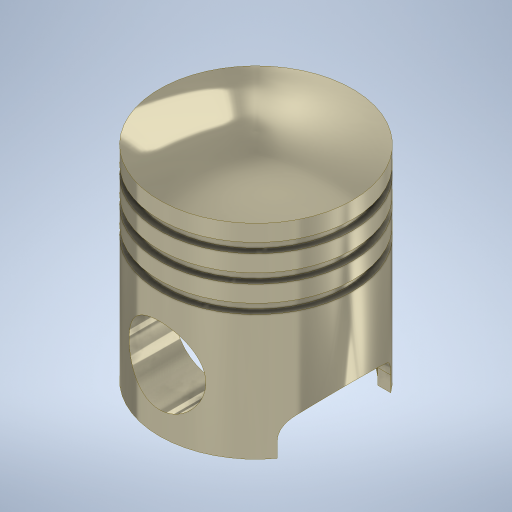
# Autodesk Inventor part: piston
Saved by Autodesk Inventor 2023 (Build 270158000, 158)
## iProperties
Created: 2023-10-20
Part Number: piston
Material: Generic
Document SubType Name: Modeling
Designer: Beatrice
Density: 1 g/cm^3
Appearance: Nickel
Author: Beatrice
Autodesk Inventor part; units mm, degrees
ref_plane "YZ Plane" through (0, 0, 0) normal (1, 0, 0) x (0, 1, 0)
sketch "Sketch1" plane through (0, 0, 0) normal (0, 0, 1) x (1, 0, 0)
  circle A0 centre (0, 0) radius 42.5
  dimension "d0" = 85
  constraints: 1 centre point, 1 coincident
  measures "d0" diameter of A0
extrude "Extrusion1" add sketch "Sketch1" along normal blind 90
ref_plane "Work Plane1" through (0, 0, 82.7) normal (0, 0, 1) x (1, 0, 0)
sketch "Sketch2" plane through (0, 0, 82.7) normal (0, 0, 1) x (1, 0, 0)
  circle A0 centre (0, 0) radius 42.5 projected
  circle A1 centre (0, 0) radius 42.5 projected
  circle A2 centre (0, 0) radius 39.5
  dimension "d4" = 79
  constraints: 3 coincident, 1 centre point
  measures "d4" diameter of A2
extrude "Extrusion2" cut sketch "Sketch2" against normal blind 4.3
pattern_linear "Rectangular Pattern1" count 3 spacing 11.6 along (0, 0, -1) of "Extrusion2"
sketch "Sketch3" plane through (0, 0, 0) normal (0, 0, -1) x (-1, 0, 0)
  circle A0 centre (0, 0) radius 38
  dimension "d10" = 76
  constraints: 1 centre point, 1 coincident
  measures "d10" diameter of A0
hole "Hole1" at (0, 0, 0) direction (0, 0, 1) diameter 76 depth 85
sketch "Sketch4" plane through (0, 0, 0) normal (0, 1, 0) x (-1, 0, 0)
  line L0 (-39.5, 78.4) -> (-39.5, 82.7) construction
  line L1 (-39.5, 82.7) -> (-42.5, 82.7) construction
  line L2 (-42.5, 82.7) -> (-42.5, 90) construction
  line L3 (-42.5, 90) -> (42.5, 90) construction
  line L4 (42.5, 90) -> (42.5, 82.7) construction
  line L5 (42.5, 82.7) -> (39.5, 82.7) construction
  line L6 (39.5, 82.7) -> (39.5, 78.4) construction
  line L7 (39.5, 78.4) -> (42.5, 78.4) construction
  line L8 (42.5, 78.4) -> (42.5, 71.1) construction
  line L9 (42.5, 71.1) -> (39.5, 71.1) construction
  line L10 (39.5, 71.1) -> (39.5, 66.8) construction
  line L11 (39.5, 66.8) -> (42.5, 66.8) construction
  line L12 (42.5, 66.8) -> (42.5, 59.5) construction
  line L13 (42.5, 59.5) -> (39.5, 59.5) construction
  line L14 (39.5, 59.5) -> (39.5, 55.2) construction
  line L15 (39.5, 55.2) -> (42.5, 55.2) construction
  line L16 (42.5, 55.2) -> (42.5, 0) construction
  line L17 (42.5, 0) -> (38, 0) construction
  line L18 (38, 0) -> (38, 85) construction
  line L19 (38, 85) -> (-38, 85) construction
  line L20 (-38, 85) -> (-38, 0) construction
  line L21 (-38, 0) -> (-42.5, 0) construction
  line L22 (-42.5, 0) -> (-42.5, 55.2) construction
  line L23 (-42.5, 55.2) -> (-39.5, 55.2) construction
  line L24 (-39.5, 55.2) -> (-39.5, 59.5) construction
  line L25 (-39.5, 59.5) -> (-42.5, 59.5) construction
  line L26 (-42.5, 59.5) -> (-42.5, 66.8) construction
  line L27 (-42.5, 66.8) -> (-39.5, 66.8) construction
  line L28 (-39.5, 66.8) -> (-39.5, 71.1) construction
  line L29 (-39.5, 71.1) -> (-42.5, 71.1) construction
  line L30 (-42.5, 71.1) -> (-42.5, 78.4) construction
  line L31 (-42.5, 78.4) -> (-39.5, 78.4) construction
  line L32 (0, -18) -> (0, 108) construction
  line L33 (-42.5, 90) -> (0, 90)
  line L34 (0, 90) -> (0, 95)
  line L35 (42.5, 90) -> (-42.5, 90) projected
  arc A0 (0, 95) -> (-42.5, 90) centre (-1.6627, -73.9918) ccw
  line L36 (0, 95) -> (-42.5, 95) construction
  point P0 (0, 0)
  dimension "d18" = 169
  dimension "d19" = 5
  constraints: 6 end point, 2 midpoint, 2 point on circle, 2 point on line, 1 centre point, 1 horizontal, 1 vertical alignment
  measures "d18" radius of A0
  measures "d19" distance of point (0, 90) L34.end
revolve "Revolution1" add sketch "Sketch4" angle 360 about axis through (0, 0, 0) along (0, 0, 1)
sketch "Sketch5" plane through (0, 0, 0) normal (0, 1, 0) x (-1, 0, 0)
  line L0 (-39.5, 78.4) -> (-39.5, 82.7) construction
  line L1 (-39.5, 82.7) -> (-42.5, 82.7) construction
  line L2 (-42.5, 82.7) -> (-42.5, 90) construction
  arc A0 (42.5, 90) -> (0, 95) centre (1.6627, -73.9918) ccw construction
  arc A1 (0, 95) -> (-42.5, 90) centre (-1.6627, -73.9918) ccw construction
  line L3 (42.5, 90) -> (42.5, 82.7) construction
  line L4 (42.5, 82.7) -> (39.5, 82.7) construction
  line L5 (39.5, 82.7) -> (39.5, 78.4) construction
  line L6 (39.5, 78.4) -> (42.5, 78.4) construction
  line L7 (42.5, 78.4) -> (42.5, 71.1) construction
  line L8 (42.5, 71.1) -> (39.5, 71.1) construction
  line L9 (39.5, 71.1) -> (39.5, 66.8) construction
  line L10 (39.5, 66.8) -> (42.5, 66.8) construction
  line L11 (42.5, 66.8) -> (42.5, 59.5) construction
  line L12 (42.5, 59.5) -> (39.5, 59.5) construction
  line L13 (39.5, 59.5) -> (39.5, 55.2) construction
  line L14 (39.5, 55.2) -> (42.5, 55.2) construction
  line L15 (42.5, 55.2) -> (42.5, 0) construction
  line L16 (42.5, 0) -> (38, 0) construction
  line L17 (38, 0) -> (38, 85) construction
  line L18 (38, 85) -> (-38, 85) construction
  line L19 (-38, 85) -> (-38, 0) construction
  line L20 (-38, 0) -> (-42.5, 0) construction
  line L21 (-42.5, 0) -> (-42.5, 55.2) construction
  line L22 (-42.5, 55.2) -> (-39.5, 55.2) construction
  line L23 (-39.5, 55.2) -> (-39.5, 59.5) construction
  line L24 (-39.5, 59.5) -> (-42.5, 59.5) construction
  line L25 (-42.5, 59.5) -> (-42.5, 66.8) construction
  line L26 (-42.5, 66.8) -> (-39.5, 66.8) construction
  line L27 (-39.5, 66.8) -> (-39.5, 71.1) construction
  line L28 (-39.5, 71.1) -> (-42.5, 71.1) construction
  line L29 (-42.5, 71.1) -> (-42.5, 78.4) construction
  line L30 (-42.5, 78.4) -> (-39.5, 78.4) construction
  line L31 (0, -108.0603) -> (0, 130.4191) construction
  circle A2 centre (0, 27) radius 16.9
  point P0 (0, 0)
  dimension "d21" = 33.8
  dimension "d22" = 27
  constraints: 1 centre point, 1 point on line
  measures "d21" diameter of A2
  measures "d22" vertical distance of L16.end A2.centre
extrude "Extrusion3" cut sketch "Sketch5" along normal through all both and the other way through all
sketch "Sketch6" plane through (0, 0, 0) normal (1, 0, 0) x (0, 1, 0)
  line L0 (-42.5, 10.1) -> (-38, 10.1) construction
  line L1 (-38, 10.1) -> (-38, 0) construction
  line L2 (-38, 0) -> (-42.5, 0) construction
  line L3 (-42.5, 0) -> (-42.5, 10.1) construction
  line L4 (38, 10.1) -> (42.5, 10.1) construction
  line L5 (42.5, 10.1) -> (42.5, 0) construction
  line L6 (42.5, 0) -> (38, 0) construction
  line L7 (38, 0) -> (38, 10.1) construction
  line L8 (-39.5, 78.4) -> (-39.5, 82.7) construction
  line L9 (-39.5, 82.7) -> (-42.5, 82.7) construction
  line L10 (-42.5, 82.7) -> (-42.5, 90) construction
  arc A0 (42.5, 90) -> (0, 95) centre (1.6627, -73.9918) ccw construction
  arc A1 (0, 95) -> (-42.5, 90) centre (-1.6627, -73.9918) ccw construction
  line L11 (42.5, 90) -> (42.5, 82.7) construction
  line L12 (42.5, 82.7) -> (39.5, 82.7) construction
  line L13 (39.5, 82.7) -> (39.5, 78.4) construction
  line L14 (39.5, 78.4) -> (42.5, 78.4) construction
  line L15 (42.5, 78.4) -> (42.5, 71.1) construction
  line L16 (42.5, 71.1) -> (39.5, 71.1) construction
  line L17 (39.5, 71.1) -> (39.5, 66.8) construction
  line L18 (39.5, 66.8) -> (42.5, 66.8) construction
  line L19 (42.5, 66.8) -> (42.5, 59.5) construction
  line L20 (42.5, 59.5) -> (39.5, 59.5) construction
  line L21 (39.5, 59.5) -> (39.5, 55.2) construction
  line L22 (39.5, 55.2) -> (42.5, 55.2) construction
  line L23 (42.5, 55.2) -> (42.5, 43.9) construction
  line L24 (42.5, 43.9) -> (38, 43.9) construction
  line L25 (38, 43.9) -> (38, 85) construction
  line L26 (38, 85) -> (-38, 85) construction
  line L27 (-38, 85) -> (-38, 43.9) construction
  line L28 (-38, 43.9) -> (-42.5, 43.9) construction
  line L29 (-42.5, 43.9) -> (-42.5, 55.2) construction
  line L30 (-42.5, 55.2) -> (-39.5, 55.2) construction
  line L31 (-39.5, 55.2) -> (-39.5, 59.5) construction
  line L32 (-39.5, 59.5) -> (-42.5, 59.5) construction
  line L33 (-42.5, 59.5) -> (-42.5, 66.8) construction
  line L34 (-42.5, 66.8) -> (-39.5, 66.8) construction
  line L35 (-39.5, 66.8) -> (-39.5, 71.1) construction
  line L36 (-39.5, 71.1) -> (-42.5, 71.1) construction
  line L37 (-42.5, 71.1) -> (-42.5, 78.4) construction
  line L38 (-42.5, 78.4) -> (-39.5, 78.4) construction
  line L39 (0, 130.4191) -> (0, -108.0603) construction
  line L40 (38, 0) -> (-38, 0) construction
  line L41 (-25, 0) -> (25, 0)
  line L42 (25, 0) -> (25, 12)
  line L43 (25, 12) -> (-25, 12) construction
  line L44 (-25, 12) -> (-25, 0)
  arc A2 (25, 12) -> (-25, 12) centre (0, -19.225) ccw
  point P0 (0, 0)
  point P1 (0, 12)
  dimension "d25" = 50
  dimension "d26" = 40
  dimension "d27" = 12
  constraints: 8 end point, 2 parallel, 2 point on circle, 2 point on line, 1 centre point, 1 horizontal, 1 midpoint, 1 perpendicular
  measures "d25" distance of L42.end L43.end
  measures "d26" radius of A2
  measures "d27" distance of L43.end L41.start
extrude "Extrusion4" cut sketch "Sketch6" along normal through all both and the other way through all
fillet "Fillet1" radius 10 4 edges at (31.4937, -25, 12) (-31.4937, -25, 12) (31.4937, 25, 12) (-31.4937, 25, 12)
ref_plane "Work Plane2" through (0, -19, 0) normal (0, 1, 0) x (-1, 0, 0)
sketch "Sketch7" plane through (0, -19, 0) normal (0, 1, 0) x (-1, 0, 0)
  line L0 (-34.6302, 78.4) -> (-34.6302, 82.7) projected
  line L1 (-34.6302, 82.7) -> (-38.0164, 82.7) projected
  line L2 (-38.0164, 82.7) -> (-38.0164, 90) projected
  line L3 (38.0164, 90) -> (38.0164, 82.7) projected
  line L4 (38.0164, 82.7) -> (34.6302, 82.7) projected
  line L5 (34.6302, 82.7) -> (34.6302, 78.4) projected
  line L6 (34.6302, 78.4) -> (38.0164, 78.4) projected
  line L7 (38.0164, 78.4) -> (38.0164, 71.1) projected
  line L8 (38.0164, 71.1) -> (34.6302, 71.1) projected
  line L9 (34.6302, 71.1) -> (34.6302, 66.8) projected
  line L10 (34.6302, 66.8) -> (38.0164, 66.8) projected
  line L11 (38.0164, 66.8) -> (38.0164, 59.5) projected
  line L12 (38.0164, 59.5) -> (34.6302, 59.5) projected
  line L13 (34.6302, 59.5) -> (34.6302, 55.2) projected
  line L14 (34.6302, 55.2) -> (38.0164, 55.2) projected
  line L15 (38.0164, 55.2) -> (38.0164, 15.9744) projected
  line L16 (38.0164, 15.9744) -> (32.909, 15.9744) projected
  line L17 (32.909, 15.9744) -> (32.909, 85) projected
  line L18 (32.909, 85) -> (-32.909, 85) projected
  line L19 (-32.909, 85) -> (-32.909, 15.9744) projected
  line L20 (-32.909, 15.9744) -> (-38.0164, 15.9744) projected
  line L21 (-38.0164, 15.9744) -> (-38.0164, 55.2) projected
  line L22 (-38.0164, 55.2) -> (-34.6302, 55.2) projected
  line L23 (-34.6302, 55.2) -> (-34.6302, 59.5) projected
  line L24 (-34.6302, 59.5) -> (-38.0164, 59.5) projected
  line L25 (-38.0164, 59.5) -> (-38.0164, 66.8) projected
  line L26 (-38.0164, 66.8) -> (-34.6302, 66.8) projected
  line L27 (-34.6302, 66.8) -> (-34.6302, 71.1) projected
  line L28 (-34.6302, 71.1) -> (-38.0164, 71.1) projected
  line L29 (-38.0164, 71.1) -> (-38.0164, 78.4) projected
  line L30 (-38.0164, 78.4) -> (-34.6302, 78.4) projected
  circle A0 centre (0, 27) radius 16.9 projected
  circle A1 centre (0, 27) radius 22.5
  point P0 (0, 0)
  dimension "d32" = 45
  constraints: 1 centre point, 1 coincident, 1 horizontal alignment
  measures "d32" diameter of A1
extrude "Extrusion5" add sketch "Sketch7" against normal up to next
mirror "Mirror1" about plane through (0, 0, 0) normal (0, 1, 0) of "Extrusion5"
body "Solid1"
